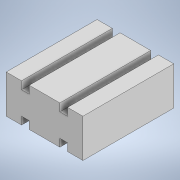
# Autodesk Inventor part: Linear Rail Carriage
Saved by Autodesk Inventor 2022 (Build 260153000, 153)
## iProperties
Created: 2021-11-30
Part Number: Linear Rail Carriage
Material: Generic
Document SubType Name: Modeling
Designer: efred
Density: 1 g/cm^3
Appearance: Default
Author: efred
Autodesk Inventor part; units mm, degrees
ref_plane "YZ Plane" through (0, 0, 0) normal (1, 0, 0) x (0, 1, 0)
ref_plane "XZ Plane" through (0, 0, 0) normal (0, 1, 0) x (-1, 0, 0)
ref_plane "XY Plane" through (0, 0, 0) normal (0, 0, 1) x (1, 0, 0)
sketch "Sketch1" plane through (0, 0, 0) normal (0, 1, 0) x (-1, 0, 0)
  line L0 (-29.8, 35.3) -> (29.8, 35.3)
  line L1 (29.8, 35.3) -> (29.8, -35.3)
  line L2 (29.8, -35.3) -> (-29.8, -35.3)
  line L3 (-29.8, -35.3) -> (-29.8, 35.3)
  line L4 (-29.8, 35.3) -> (29.8, -35.3) construction
  line L5 (29.8, 35.3) -> (-29.8, -35.3) construction
  point P0 (0, 0)
  dimension "d0" = 70.6
  dimension "d1" = 59.6
  constraints: 12 end point, 2 midpoint, 2 parallel, 1 horizontal, 1 perpendicular
  measures "d0" distance of L2.end L0.start
  measures "d1" distance of L1.end L2.end
extrude "Extrusion1" add sketch "Sketch1" along normal mid plane 29.8
sketch "Sketch2" plane through (0, 14.9, 0) normal (0, 1, 0) x (1, 0, 0)
  line L0 (-29.8, -35.3) -> (29.8, -35.3) projected
  line L1 (29.8, 35.3) -> (-29.8, 35.3) projected
  line L2 (-17.9, -35.3) -> (-11.9, -35.3)
  line L3 (-11.9, -35.3) -> (-11.9, 35.3)
  line L4 (-11.9, 35.3) -> (-17.9, 35.3)
  line L5 (-17.9, 35.3) -> (-17.9, -35.3)
  line L6 (11.9, -35.3) -> (17.9, -35.3)
  line L7 (17.9, -35.3) -> (17.9, 35.3)
  line L8 (17.9, 35.3) -> (11.9, 35.3)
  line L9 (11.9, 35.3) -> (11.9, -35.3)
  line L10 (-29.8, 35.3) -> (-29.8, -35.3) projected
  line L11 (0, -35.3) -> (0, 35.3) construction
  point P0 (0, 0)
  dimension "d4" = 6
  dimension "d5" = 11.9
  constraints: 18 end point, 4 parallel, 4 point on line, 2 horizontal, 2 midpoint, 2 perpendicular, 2 other
  measures "d4" distance between parallel lines of L3 L5
  measures "d5" distance between parallel lines of L10 L5
extrude "Extrusion2" cut sketch "Sketch2" against normal blind 6 contours L5 L1 L3 L0 | L9 L1 L7 L0
mirror "Mirror1" about plane through (0, 0, 0) normal (0, 1, 0) of "Extrusion2"
body "Solid1"
